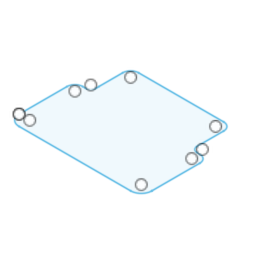
base v1 (Autodesk Fusion 360 design; units mm, degrees)
Autodesk Fusion 360 part; units mm, degrees
sketch "Boceto1" plane through (0, 0, 0) normal (1, 0, 0) x (0, 1, 0)
  line L0 (0, 0) -> (20, 0)
  line L1 (20, 0) -> (20, 77)
  line L2 (0, 0) -> (0, 124.8471)
  line L3 (20, 77) -> (20, 105.1035)
  line L4 (20, 105.1035) -> (0, 124.8471)
  dimension "d1" = 20
  dimension "d3" = 77
  constraint coincident L0.start L2.start
  constraint horizontal L0
  constraint perpendicular L0 L2
  constraint parallel L1 L3
  measures "d1" distance of L0.start L0.end
  measures "d3" distance of L0.end L1.end
extrude "Extruir1" add sketch "Boceto1" along normal blind 10 makes body 1
sketch "Boceto2" plane through (0, 0, 0) normal (1, 0, 0) x (0, 1, 0)
  line L0 (20, 77) -> (98, 0)
  line L1 (0, 96.7436) -> (0, 125)
  line L2 (0, 125) -> (125, 0)
  line L3 (125, 0) -> (98, 0)
  line L4 (20, 77) -> (0, 96.7436)
  constraint parallel L0 L4
extrude "Extruir2" add sketch "Boceto2" against normal blind 10 separate body makes body 2
copy_body "CopiarPegarCuerpos1" bodies 2 1 makes body 3 makes body 4
move_body "Desplazar1" bodies 3 4 to x (1, 0, 0) y (0, 1, 0) z (0, 0, 1) at (60, 0, 0)
move_body "Desplazar2" bodies 3 to x (1, 0, 0) y (0, 1, 0) z (0, 0, 1) at (20, 0, 0)
move_body "Desplazar3" bodies 4 3 to x (1, 0, 0) y (0, 1, 0) z (0, 0, 1) at (-10, 0, 0)
move_body "Desplazar4" bodies 2 1 4 3 to x (1, 0, 0) y (0, 1, 0) z (0, 0, 1) at (-30, 0, 0)
hole "Agujero1" at (-30, 9.7138, 57.6289) direction (1, 0, 0) diameter 5 end through all bodies 4 1
sketch "Boceto4" plane through (-30, 0, 0) normal (-1, 0, 0) x (0, -1, 0)
  circle A0 centre (-9.7138, 57.6289) radius 2.5
  line L0 (-20, 0) -> (0, 0)
  line L1 (0, 0) -> (0, 124.8471)
  line L2 (0, 124.8471) -> (-20, 105.1035)
  line L3 (-20, 105.1035) -> (-20, 0)
  circle A1 centre (-9.7138, 57.6289) radius 2.5
  constraint concentric A0 A1
extrude "Extruir3" add sketch "Boceto4" along normal blind 65 separate body contours A0 A1 makes body 5
move_body "Desplazar5" bodies 5 to x (1, 0, 0) y (0, 1, 0) z (0, 0, 1) at (62.5, 0, 0)
sketch "Boceto5" plane through (-30, 0, 0) normal (-1, 0, 0) x (0, -1, 0)
  circle A0 centre (-9.7138, 57.6289) radius 2.5
  line L0 (-20, 0) -> (0, 0)
  line L1 (0, 0) -> (0, 124.8471)
  line L2 (0, 124.8471) -> (-20, 105.1035)
  line L3 (-20, 105.1035) -> (-20, 0)
  line L4 (-9.7138, 57.6289) -> (-9.7138, 60.1289)
  line L5 (-9.7138, 57.6289) -> (-7.2138, 57.6289)
  line L6 (-9.7138, 57.6289) -> (-9.7138, 60.1289)
  line L7 (-7.946, 59.3967) -> (-9.7138, 57.6289)
  line L8 (-9.7138, 57.6289) -> (-7.946, 59.3967)
  line L9 (0, 0) -> (120, 0)
  line L10 (120, 0) -> (156.825, 0)
  line L11 (-7.946, 59.3967) -> (-7.946, 0)
  constraint coincident A0.centre L4.start
  constraint coincident A0 L4.end
  constraint vertical L4
  constraint coincident A0 L5.end
  constraint perpendicular L4 L5
  constraint coincident A0 L7.start
  constraint coincident L0.end L1.start
  constraint perpendicular L1 L9
  constraint perpendicular L1 L10
  constraint coincident L0 L11.end
  constraint perpendicular L0 L11
sketch "Boceto7" plane through (0, 0, 0) normal (0, 0, 1) x (1, 0, 0)
  line L0 (-124.6984, 19.9078) -> (-124.6984, 110)
  line L1 (-104.6984, 125) -> (-109.6984, 125)
  line L2 (125.3016, 19.9078) -> (125.3016, 110)
  line L3 (-94.6984, 140) -> (-94.6984, 185)
  line L4 (95.3016, 135) -> (95.3016, 185)
  line L5 (105.3016, 125) -> (110.3016, 125)
  line L6 (-79.6984, 200) -> (80.3016, 200)
  line L7 (-104.6984, 0) -> (105.3016, 0)
  line L8 (125.3016, 20) -> (125.3016, 19.9078)
  arc A0 (-79.6984, 200) -> (-94.6984, 185) centre (-79.6984, 185) ccw
  arc A1 (95.3016, 185) -> (80.3016, 200) centre (80.3016, 185) ccw
  arc A2 (-109.6984, 125) -> (-124.6984, 110) centre (-109.6984, 110) ccw
  arc A3 (125.3016, 110) -> (110.3016, 125) centre (110.3016, 110) ccw
  arc A4 (95.3016, 135) -> (105.3016, 125) centre (105.3016, 135) ccw
  line L9 (-94.6984, 140) -> (-94.6984, 135)
  arc A5 (-104.6984, 125) -> (-94.6984, 135) centre (-104.6984, 135) ccw
  arc A6 (105.3016, 0) -> (125.3016, 20) centre (105.3016, 20) ccw
  arc A7 (-124.6984, 20) -> (-104.6984, 0) centre (-104.6984, 20) ccw
  dimension "d82" = 15
  dimension "d83" = 15
  dimension "d84" = 15
  dimension "d86" = 15
  dimension "d87" = 10
  dimension "d88" = 10
  dimension "d90" = 20
  dimension "d91" = 20
  constraint perpendicular L0 L1
  constraint perpendicular L4 L6
  constraint perpendicular L2 L7
  constraint tangent L3 A0
  constraint tangent L6 A0
  constraint tangent L4 A1
  constraint tangent L6 A1
  constraint tangent L0 A2
  constraint tangent L1 A2
  constraint tangent L2 A3
  constraint tangent L4 A4
  constraint tangent L5 A4
  constraint perpendicular L1 L9
  constraint tangent L1 A5
  constraint tangent L9 A5
  constraint tangent L7 A6
  constraint tangent L8 A6
  measures "d82" radius of A0
  measures "d83" radius of A1
  measures "d84" radius of A2
  measures "d86" radius of A3
  measures "d87" radius of A4
  measures "d88" radius of A5
  measures "d90" radius of A6
  measures "d91" radius of A7
move_body "Desplazar6" bodies 2 1 to x (1, 0, 0) y (0, 1, 0) z (0, 0, 1) at (-10, 0, 0)
move_body "Desplazar7" bodies 4 3 to x (1, 0, 0) y (0, 1, 0) z (0, 0, 1) at (10, 0, 0)
move_face "MoveFace1" by (9, 0, 0) 1 faces at (32.5, 8.963, 57.2674) on bodies 5
move_face "MoveFace2" by (-11, 0, 0) 1 faces at (-32.5, 8.963, 57.9905) on bodies 5
move_body "Desplazar8" bodies 2 1 to x (1, 0, 0) y (0, 1, 0) z (0, 0, 1) at (-10, 0, 0)
move_body "Desplazar9" bodies 4 3 to x (1, 0, 0) y (0, 1, 0) z (0, 0, 1) at (10, 0, 0)
move_body "Desplazar10" bodies 5 to x (1, 0, 0) y (0, 1, 0) z (0, 0, 1) at (10, 0, 0)
move_face "MoveFace3" by (-18, 0, 0) 1 faces at (-33.5, 8.963, 57.9905) on bodies 5
sketch "Boceto12" plane through (0, 0, 0) normal (1, 0, 0) x (0, 1, 0)
  line L0 (0, 0) -> (0, 125)
  line L1 (0, 0) -> (20.175, 0)
  line L2 (20.175, 0) -> (20.175, 105.0001)
  line L3 (0, 125) -> (20.175, 105.0001)
  dimension "d45" = 125
  dimension "d54" = 20.175
  constraint vertical L0
  constraint coincident L0.start L1.start
  constraint vertical L2
  constraint perpendicular L1 L2
  measures "d45" distance of L0.start L0.end
  measures "d54" distance of L0.start L1.end
sketch "Boceto13" plane through (0, 0, 0) normal (1, 0, 0) x (0, 1, 0)
  line L0 (98.4379, 0) -> (127.2254, 0)
  line L1 (0, 125) -> (0, 96.716)
  line L2 (0, 96.716) -> (98.4379, 0)
  line L3 (0, 125) -> (127.2254, 0)
  line L4 (98.4379, 0) -> (127.2254, 0)
  dimension "d51" = 28.284
  dimension "d52" = 138
  constraint vertical L1
  constraint parallel L2 L3
  measures "d51" distance of L1.start L1.end
  measures "d52" distance of L1.end L0.start
extrude "Extruir4" add sketch "Boceto12" along normal blind 10 separate body makes body 6
extrude "Extruir5" add sketch "Boceto13" against normal blind 10 separate body makes body 7
copy_body "CopiarPegarCuerpos2" bodies 7 6 makes body 8 makes body 9
move_body "Desplazar11" bodies 8 9 to x (1, 0, 0) y (0, 1, 0) z (0, 0, 1) at (-20, 0, 0)
move_body "Desplazar12" bodies 7 6 to x (1, 0, 0) y (0, 1, 0) z (0, 0, 1) at (20, 0, 0)
move_body "Desplazar13" bodies 9 8 to x (1, 0, 0) y (0, 1, 0) z (0, 0, 1) at (-30, 0, 0)
move_body "Desplazar14" bodies 7 6 to x (1, 0, 0) y (0, 1, 0) z (0, 0, 1) at (30, 0, 0)
move_body "Desplazar15" bodies 7 to x (1, 0, 0) y (0, 1, 0) z (0, 0, 1) at (20, 0, 0)
move_body "Desplazar16" bodies 6 to x (1, 0, 0) y (0, 1, 0) z (0, 0, 1) at (-10, 0, 0)
move_body "Desplazar17" bodies 7 to x (1, 0, 0) y (0, 1, 0) z (0, 0, 1) at (-10, 0, 0)
extrude "Extruir6" add sketch "Boceto7" against normal blind 3 separate body makes body 10
move_body "Desplazar18" bodies 8 9 to x (1, 0, 0) y (0, 1, 0) z (0, 0, 1) at (10, 0, 0)
move_body "Desplazar19" bodies 6 7 to x (1, 0, 0) y (0, 1, 0) z (0, 0, 1) at (-10, 0, 0)
sketch "Boceto19" plane through (-40, 0, 0) normal (-1, 0, 0) x (0, -1, 0)
  line L0 (-20.175, 0) -> (0, 0)
  line L1 (0, 0) -> (0, 125)
  line L2 (0, 125) -> (-20.175, 105.0001)
  line L3 (-20.175, 105.0001) -> (-20.175, 0)
  line L4 (-200, 0) -> (-200, 63)
  line L5 (0, 0) -> (0, 33)
  dimension "d104" = 63
  dimension "d105" = 33
  constraint vertical L4
  constraint coincident L0.end L1.start
  constraint perpendicular L0 L5
  measures "d104" distance of L4.start L4.end
  measures "d105" distance of L0.end L5.end
sketch "Boceto20" plane through (0, 0, 0) normal (1, 0, 0) x (0, 1, 0)
sketch "Boceto21" plane through (0, 0, -3) normal (0, 0, -1) x (1, 0, 0)
  line L0 (-109.6984, -125) -> (-104.6984, -125)
  arc A0 (-94.6984, -135) -> (-104.6984, -125) centre (-104.6984, -135) ccw
  line L1 (-94.6984, -135) -> (-94.6984, -185)
  arc A1 (-94.6984, -185) -> (-79.6984, -200) centre (-79.6984, -185) ccw
  line L2 (-79.6984, -200) -> (80.3016, -200)
  arc A2 (80.3016, -200) -> (95.3016, -185) centre (80.3016, -185) ccw
  line L3 (95.3016, -185) -> (95.3016, -135)
  arc A3 (105.3016, -125) -> (95.3016, -135) centre (105.3016, -135) ccw
  line L4 (105.3016, -125) -> (110.3016, -125)
  arc A4 (110.3016, -125) -> (125.3016, -110) centre (110.3016, -110) ccw
  line L5 (125.3016, -110) -> (125.3016, -20)
  arc A5 (125.3016, -20) -> (105.3016, 0) centre (105.3016, -20) ccw
  line L6 (105.3016, 0) -> (-104.6984, 0)
  arc A6 (-104.6984, 0) -> (-124.6984, -20) centre (-104.6984, -20) ccw
  line L7 (-124.6984, -20) -> (-124.6984, -110)
  arc A7 (-124.6984, -110) -> (-109.6984, -125) centre (-109.6984, -110) ccw
  line L8 (-94.6984, -185) -> (-84.6984, -185)
  line L9 (-84.6984, -199.1421) -> (-84.6984, -169.1421)
  line L10 (95.3016, -185) -> (85.3016, -185)
  line L11 (85.3016, -199.1421) -> (85.3016, -169.1421)
  dimension "d106" = 10
  dimension "d107" = 30
  dimension "d108" = 10
  dimension "d109" = 30
  constraint coincident L1.end A1.start
  constraint perpendicular L1 L8
  constraint coincident A1 L9.start
  constraint perpendicular L8 L9
  constraint coincident A2.end L3.start
  constraint perpendicular L3 L10
  constraint coincident A2 L11.start
  constraint perpendicular L10 L11
  measures "d106" distance of L1.end L8.end
  measures "d107" distance of L9.start L9.end
  measures "d108" distance of A2.end L10.end
  measures "d109" distance of L11.start L11.end
sketch "Boceto22" plane through (-40, 0, 0) normal (-1, 0, 0) x (0, -1, 0)
  line L0 (-199.9174, -16.3413) -> (-169.9174, -16.3413)
  circle A0 centre (-169.9174, -16.3413) radius 13
  dimension "d110" = 30
  dimension "d111" = 26
  constraint horizontal L0
  constraint coincident L0.end A0.centre
  measures "d110" distance of L0.start L0.end
  measures "d111" diameter of A0
sketch "Boceto23" plane through (-40, 0, 0) normal (-1, 0, 0) x (0, -1, 0)
  circle A0 centre (-169.8636, -16.3266) radius 7.5
  dimension "d122" = 15
  measures "d122" diameter of A0
extrude "Extruir7" add sketch "Boceto22" against normal blind 50 separate body makes body 11
sketch "Boceto24" plane through (0, 0, 0) normal (0, 1, 0) x (1, 0, 0)
  line L0 (-125, 0) -> (-115, 0)
  dimension "d114" = 10
  constraint horizontal L0
  measures "d114" distance of L0.start L0.end
move_body "Desplazar20" bodies 11 to x (1, 0, 0) y (0, 1, 0) z (0, 0, 1) at (-75, 0, 0)
copy_body "CopiarPegarCuerpos3" bodies 11 makes body 12
move_body "Desplazar21" bodies 12 to x (1, 0, 0) y (0, 1, 0) z (0, 0, 1) at (180, 0, 0)
sketch "Boceto25" plane through (0, 0, 0) normal (1, 0, 0) x (0, 1, 0)
  circle A0 centre (169.891, -16.3851) radius 7.5
  dimension "d121" = 15
  measures "d121" diameter of A0
extrude "Extruir8" add sketch "Boceto23" along normal blind 20 separate body makes body 13
move_body "Desplazar22" bodies 13 to x (1, 0, 0) y (0, 1, 0) z (0, 0, 1) at (-75, 0, 0)
move_body "Desplazar23" bodies 11 13 to x (1, 0, 0) y (0, 1, 0) z (0, 0, 1) at (40, 0, 0)
copy_body "CopiarPegarCuerpos4" bodies 13 makes body 14
move_body "Desplazar24" bodies 14 to x (1, 0, 0) y (0, 1, 0) z (0, 0, 1) at (210, 0, 0)
move_body "Desplazar25" bodies 14 12 to x (1, 0, 0) y (0, 1, 0) z (0, 0, 1) at (-40, 0, 0)
move_body "Desplazar26" bodies 14 12 11 13 to x (1, 0, 0) y (0, 1, 0) z (0, 0, 1) at (0, 15, 0)
sketch "Boceto26" plane through (-40, 0, 0) normal (-1, 0, 0) x (0, -1, 0)
  circle A0 centre (-184.9222, -16.7336) radius 32.5
  dimension "d140" = 65
  measures "d140" diameter of A0
extrude "Extruir9" add sketch "Boceto26" along normal blind 25 separate body makes body 15
move_body "Desplazar27" bodies 15 to x (1, 0, 0) y (0, 1, 0) z (0, 0, 1) at (-55, 0, 0)
copy_body "CopiarPegarCuerpos5" bodies 15 makes body 16
move_body "Desplazar28" bodies 16 to x (1, 0, 0) y (0, 1, 0) z (0, 0, 1) at (215, 0, 0)
move_body "Desplazar29" bodies 9 8 10 6 5 7 11 13 15 12 14 16 to x (1, 0, 0) y (0, 1, 0) z (0, 0, 1) at (0, 0, 65)
move_body "Desplazar30" bodies 16 14 12 11 13 15 to x (1, 0, 0) y (0, 1, 0) z (0, 0, 1) at (0, -20, 0)
move_body "Desplazar31" bodies 11 13 15 12 14 16 to x (1, 0, 0) y (0, 1, 0) z (0, 0, 1) at (0, 0, -10)
move_body "Desplazar32" bodies 15 10 8 7 5 9 6 13 11 12 14 16 to x (1, 0, 0) y (0, 0.984808, 0.173648) z (0, -0.173648, 0.984808) at (0, 13.7327, -31.1327)
move_body "Desplazar33" bodies 15 8 5 10 6 7 9 11 13 12 14 16 to x (1, 0, 0) y (0, 1, 0) z (0, 0, 1) at (0, 0, -3)
sketch "Boceto27" plane through (0, 0, 0) normal (1, 0, 0) x (0, 1, 0)
  line L0 (-105.1222, 0) -> (-150, 0)
  line L1 (-150, 0) -> (-105.1222, 0) construction
  line L2 (-150, 0) -> (-135.1222, 1.9111)
  line L3 (-135.1222, 0) -> (-105.1222, 0)
  line L4 (-105.1222, 0) -> (54.2264, 92)
  line L5 (54.2264, 92) -> (46.7264, 104.9904)
  line L6 (46.7264, 104.9904) -> (-130.8651, 2.4579)
  line L7 (-150, 0) -> (-130.8651, 2.4579)
  dimension "d171" = 15
  dimension "d172" = 30
  dimension "d173" = 184
  dimension "d175" = 15
  constraint horizontal L0
  constraint horizontal L1
  constraint coincident L1 L3.start
  constraint perpendicular L4 L5
  constraint perpendicular L5 L6
  constraint parallel L2 L7
  measures "d171" distance of L0.end L2.end
  measures "d172" distance of L3.start L0.start
  measures "d173" distance of L0.start L4.end
  measures "d175" distance of L4.end L5.end
extrude "Extruir10" add sketch "Boceto27" along normal blind 10 separate body makes body 17
copy_body "CopiarPegarCuerpos6" bodies 17 makes body 18
move_body "Desplazar34" bodies 18 to x (1, 0, 0) y (0, 1, 0) z (0, 0, 1) at (-30, 0, 0)
move_body "Desplazar35" bodies 17 to x (1, 0, 0) y (0, 1, 0) z (0, 0, 1) at (20, 0, 0)
sketch "Boceto28" plane through (0, 0, 0) normal (0, 1, 0) x (1, 0, 0)
sketch "Boceto29" plane through (0, 0, 0) normal (1, 0, 0) x (0, 1, 0)
extrude "Extruir11" add sketch "Boceto27" along normal blind 30 separate body makes body 19
move_body "Desplazar36" bodies 19 to x (1, 0, 0) y (0, 1, 0) z (0, 0, 1) at (40, 0, 0)
move_body "Desplazar37" bodies 19 to x (1, 0, 0) y (0, 1, 0) z (0, 0, 1) at (10, 0, 0)
move_body "Desplazar38" bodies 19 to x (1, 0, 0) y (0, 1, 0) z (0, 0, 1) at (-10, 0, 0)
move_face "MoveFace4" by (0, -70, 0) 1 faces at (50, 51.7264, 96.3301) on bodies 19
move_body "Desplazar39" bodies 19 to x (1, 0, 0) y (0, 1, 0) z (0, 0, 1) at (-10, 0, 0)
move_face "MoveFace5" by (60, 0, 0) 1 faces at (60, -80.5869, 25.7125) on bodies 19
move_face "MoveFace6" by (0, 0, -60) 1 faces at (60, -69.506, 20.563) on bodies 19
hidden bodies 1 2 3 4 5 19
named bodies: "soporte recto izq", "soporte incl izq", "soporte incl der", "soporte recto der", "tope flipper", "soporte recto der v1", "soporte incl der v1", "soporte incl izq v1", "soporte recto izq v1", "soporte incl izq v1", "soporte recto izq v1", "motor izq", "motor der", "rueda izq", "rueda der"
